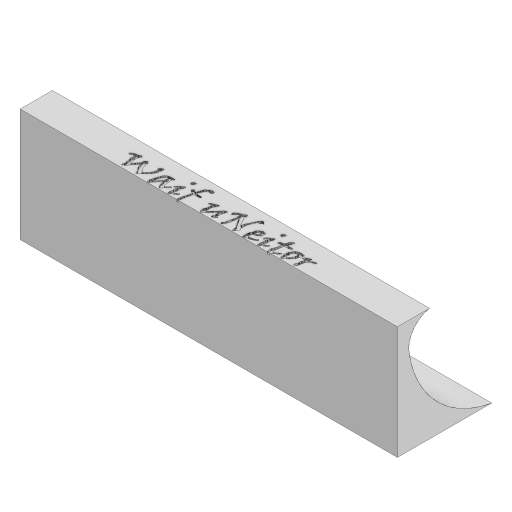
# Autodesk Inventor part: aaaaaa
Saved by Autodesk Inventor 2024.3 (Build 283343000, 343)
## iProperties
Created: 2025-09-24
Part Number: aaaaaa
Material: Generic
Document SubType Name: Modeling
Designer: danie
Density: 1 g/cm^3
Appearance: Default
Author: danie
Autodesk Inventor part; units mm, degrees
(part 1 of 3)
ref_plane "YZ Plane" through (0, 0, 0) normal (1, 0, 0) x (0, 1, 0)
ref_plane "XZ Plane" through (0, 0, 0) normal (0, 1, 0) x (-1, 0, 0)
ref_plane "XY Plane" through (0, 0, 0) normal (0, 0, 1) x (1, 0, 0)
sketch "Sketch1" plane through (0, 0, 0) normal (0, 1, 0) x (-1, 0, 0)
  line L0 (0, 0) -> (200, 0)
  line L1 (200, 0) -> (200, -50)
  line L2 (200, -50) -> (0, -50)
  line L3 (0, -50) -> (0, 0)
  dimension "d0" = 200
  dimension "d1" = 50
  constraints: 8 end point, 2 parallel, 1 horizontal, 1 perpendicular
  measures "d0" distance of L1.end L2.end
  measures "d1" distance of L0.end L1.end
extrude "Extrusion1" add sketch "Sketch1" along normal blind 60
sketch "Sketch2" plane through (0, 0, 0) normal (1, 0, 0) x (0, 0, -1)
  line L0 (0, 0) -> (10, 0)
  line L1 (50, 0) -> (0, 0) projected
  line L2 (10, 0) -> (10, 42.4907)
  line L3 (50, 60) -> (0, 60) projected
  line L4 (0, 60) -> (10, 60)
  line L5 (0, 60) -> (0, 0)
  line L6 (50, 0) -> (50, 60) projected
  line L7 (50, 0) -> (10, 0)
  line L8 (10, 36.0626) -> (10, 0)
  line L9 (50, 0) -> (10, 0)
  line L10 (10, 0) -> (10, 60)
  line L11 (50, 0) -> (5.9553, 46.7873)
  line L12 (5.9553, 46.7873) -> (5.9553, 0)
  line L13 (5.9553, 0) -> (5.9553, 60)
  arc A0 (5.9553, 46.7873) -> (50, 0) centre (58.9478, 52.5484) ccw
  arc A1 (21.7431, 60) -> (5.9553, 46.7873) centre (19.3779, 46.7873) ccw
  line L14 (10, 60) -> (50, 60)
  line L15 (50, 60) -> (50, 0)
  point P0 (17.0127, 60)
  dimension "d4" = 10
  constraints: 26 end point, 7 collinear, 7 point on line, 4 point on circle, 3 perpendicular, 2 centre point, 1 tangent
  measures "d4" distance of L0.start L0.end
extrude "Extrusion2" cut sketch "Sketch2" against normal blind 205.75 contours A1 L10 L11 | L11 L2 A0 | L11 L10 A1 L3 L6 | A0 L2 L11
sketch "Sketch3" plane through (0, 60, 0) normal (0, 1, 0) x (1, 0, 0)
  line L0 (-151.1336, 0) -> (-72.8185, 0)
  line L1 (-200, 0) -> (0, 0) projected
  line L2 (-151.1336, 0) -> (-151.1336, 4.8193)
  line L3 (-151.1336, 1.3121) -> (-68.8391, 1.3121)
  spline S0 degree 2 poles (-146.2846, 10.7529) (-145.9785, 10.6182) (-145.8927, 10.508) knots 0 0 0 1 1 1
  line L4 (-145.8927, 10.508) -> (-145.8683, 10.2753)
  line L5 (-145.8683, 10.2753) -> (-145.5376, 10.2019)
  spline S1 degree 2 poles (-145.5376, 10.2019) (-145.5989, 10.1284) (-146.0029, 9.81) knots 0 0 0 1 1 1
  line L6 (-146.0029, 9.81) -> (-146.1499, 9.4549)
  line L7 (-146.1499, 9.4549) -> (-146.1499, 9.259)
  line L8 (-146.1499, 9.259) -> (-146.1009, 9.1121)
  line L9 (-146.1009, 9.1121) -> (-146.3458, 8.6468)
  line L10 (-146.3458, 8.6468) -> (-146.3213, 8.1447)
  line L11 (-146.3213, 8.1447) -> (-146.4193, 7.8998)
  line L12 (-146.4193, 7.8998) -> (-146.5295, 7.2019)
  line L13 (-146.5295, 7.2019) -> (-146.4193, 6.9815)
  line L14 (-146.4193, 6.9815) -> (-146.456, 6.7121)
  line L15 (-146.456, 6.7121) -> (-146.4193, 6.6386)
  line L16 (-146.4193, 6.6386) -> (-146.5295, 6.5651)
  line L17 (-146.5295, 6.5651) -> (-146.1744, 5.2549)
  line L18 (-146.1744, 5.2549) -> (-146.2601, 5.1937)
  line L19 (-146.2601, 5.1937) -> (-145.758, 4.3121)
  line L20 (-145.758, 4.3121) -> (-145.5376, 4.4223)
  line L21 (-145.5376, 4.4223) -> (-145.5131, 4.557)
  spline S2 degree 2 poles (-145.5131, 4.557) (-145.5131, 4.6182) (-145.3662, 4.8141) (-145.1213, 5.01) knots 0 0 0 1 2 2 2
  spline S3 degree 2 poles (-145.1213, 5.01) (-145.1213, 5.0835) (-144.9009, 5.4019) knots 0 0 0 1 1 1
  line L22 (-144.9009, 5.4019) -> (-144.8764, 5.3774)
  line L23 (-144.8764, 5.3774) -> (-144.7662, 5.4753)
  line L24 (-144.7662, 5.4753) -> (-144.7295, 5.61)
  line L25 (-144.7295, 5.61) -> (-144.5948, 5.7325)
  line L26 (-144.5948, 5.7325) -> (-144.6193, 5.9651)
  spline S4 degree 2 poles (-144.6193, 5.9651) (-144.5091, 5.9896) (-144.2029, 6.1488) knots 0 0 0 1 1 1
  line L27 (-144.2029, 6.1488) -> (-144.1172, 6.308)
  line L28 (-144.1172, 6.308) -> (-144.056, 6.308)
  spline S5 degree 2 poles (-144.056, 6.308) (-143.9336, 6.5406) (-143.7009, 6.7121) knots 0 0 0 1 1 1
  line L29 (-143.7009, 6.7121) -> (-143.6764, 6.8835)
  spline S6 degree 2 poles (-143.6764, 6.8835) (-143.6029, 6.9447) (-143.3213, 7.3121) knots 0 0 0 1 1 1
  line L30 (-143.3213, 7.3121) -> (-143.3458, 7.3488)
  line L31 (-143.3458, 7.3488) -> (-143.2601, 7.4223)
  line L32 (-143.2601, 7.4223) -> (-143.2601, 7.7039)
  line L33 (-143.2601, 7.7039) -> (-143.1499, 8.059)
  line L34 (-143.1499, 8.059) -> (-143.2846, 8.3406)
  line L35 (-143.2846, 8.3406) -> (-143.2601, 8.6223)
  line L36 (-143.2601, 8.6223) -> (-143.3458, 8.7815)
  spline S7 degree 2 poles (-143.3458, 8.7815) (-143.3336, 8.8427) (-143.1744, 9.0019) knots 0 0 0 1 1 1
  line L37 (-143.1744, 9.0019) -> (-143.0642, 9.0019)
  line L38 (-143.0642, 9.0019) -> (-142.8683, 9.1121)
  line L39 (-142.8683, 9.1121) -> (-142.8683, 9.3202)
  line L40 (-142.8683, 9.3202) -> (-142.6846, 9.4182)
  line L41 (-142.6846, 9.4182) -> (-142.5376, 9.357)
  spline S8 degree 2 poles (-142.5376, 9.357) (-142.4274, 9.5406) (-142.3417, 9.6386) knots 0 0 0 1 1 1
  line L42 (-142.3417, 9.6386) -> (-141.9866, 9.7488)
  line L43 (-141.9866, 9.7488) -> (-141.705, 9.6019)
  line L44 (-141.705, 9.6019) -> (-141.5091, 9.0019)
  line L45 (-141.5091, 9.0019) -> (-141.1295, 8.757)
  line L46 (-141.1295, 8.757) -> (-141.0683, 7.9488)
  line L47 (-141.0683, 7.9488) -> (-141.0315, 7.8019)
  line L48 (-141.0315, 7.8019) -> (-141.0683, 7.6182)
  line L49 (-141.0683, 7.6182) -> (-140.958, 7.5202)
  line L50 (-140.958, 7.5202) -> (-140.8846, 7.0672)
  line L51 (-140.8846, 7.0672) -> (-140.7131, 6.5039)
  line L52 (-140.7131, 6.5039) -> (-140.6764, 6.308)
  line L53 (-140.6764, 6.308) -> (-140.0152, 4.9733)
  line L54 (-140.0152, 4.9733) -> (-139.5866, 4.2386)
  line L55 (-139.5866, 4.2386) -> (-139.2927, 4.1406)
  line L56 (-139.2927, 4.1406) -> (-139.256, 3.7611)
  line L57 (-139.256, 3.7611) -> (-139.0968, 3.6753)
  line L58 (-139.0968, 3.6753) -> (-139.0111, 3.6753)
  line L59 (-139.0111, 3.6753) -> (-138.8397, 3.5039)
  spline S9 degree 2 poles (-138.8397, 3.5039) (-138.7662, 3.4304) (-138.5948, 3.1121) knots 0 0 0 1 1 1
  line L60 (-138.5948, 3.1121) -> (-138.3744, 3.1488)
  line L61 (-138.3744, 3.1488) -> (-138.2764, 3.357)
  line L62 (-138.2764, 3.357) -> (-138.1295, 3.4549)
  line L63 (-138.1295, 3.4549) -> (-138.0315, 3.6019)
  spline S10 degree 2 poles (-138.0315, 3.6019) (-137.9825, 3.6753) (-137.7376, 3.8957) knots 0 0 0 1 1 1
  line L64 (-137.7376, 3.8957) -> (-137.6764, 3.9202)
  line L65 (-137.6764, 3.9202) -> (-137.5172, 4.1284)
  spline S11 degree 2 poles (-137.5172, 4.1284) (-137.4315, 4.2386) (-137.2601, 4.3366) knots 0 0 0 1 1 1
  line L66 (-137.2601, 4.3366) -> (-137.2111, 4.4835)
  line L67 (-137.2111, 4.4835) -> (-137.0029, 4.6672)
  spline S12 degree 2 poles (-137.0029, 4.6672) (-136.8805, 4.9488) (-136.7213, 5.0835) (-136.5376, 5.157) knots 0 0 0 1 2 2 2
  line L68 (-136.5376, 5.157) -> (-136.4764, 5.3284)
  line L69 (-136.4764, 5.3284) -> (-136.4397, 5.3039)
  line L70 (-136.4397, 5.3039) -> (-136.354, 5.6223)
  spline S13 degree 2 poles (-136.354, 5.6223) (-136.3417, 5.6713) (-136.207, 5.8672) knots 0 0 0 1 1 1
  line L71 (-136.207, 5.8672) -> (-136.1213, 5.8672)
  line L72 (-136.1213, 5.8672) -> (-136.0111, 5.9651)
  line L73 (-136.0111, 5.9651) -> (-135.9499, 6.2835)
  line L74 (-135.9499, 6.2835) -> (-135.705, 6.7488)
  line L75 (-135.705, 6.7488) -> (-135.5948, 6.8468)
  line L76 (-135.5948, 6.8468) -> (-135.6683, 6.9447)
  line L77 (-135.6683, 6.9447) -> (-135.5213, 7.2264)
  line L78 (-135.5213, 7.2264) -> (-135.5213, 7.7039)
  line L79 (-135.5213, 7.7039) -> (-135.4601, 7.7039)
  line L80 (-135.4601, 7.7039) -> (-135.3744, 7.8019)
  line L81 (-135.3744, 7.8019) -> (-135.3131, 7.8019)
  line L82 (-135.3131, 7.8019) -> (-135.3744, 8.3406)
  line L83 (-135.3744, 8.3406) -> (-135.4601, 8.757)
  line L84 (-135.4601, 8.757) -> (-135.9866, 8.757)
  line L85 (-135.9866, 8.757) -> (-136.1213, 9.0386)
  line L86 (-136.1213, 9.0386) -> (-136.0111, 9.1733)
  line L87 (-136.0111, 9.1733) -> (-135.9499, 9.3202)
  line L88 (-135.9499, 9.3202) -> (-135.8274, 9.4549)
  spline S14 degree 2 poles (-135.8274, 9.4549) (-135.7662, 9.5284) (-135.705, 9.6998) knots 0 0 0 1 1 1
  line L89 (-135.705, 9.6998) -> (-135.5703, 9.7855)
  line L90 (-135.5703, 9.7855) -> (-135.5703, 9.9202)
  line L91 (-135.5703, 9.9202) -> (-135.3744, 10.0304)
  line L92 (-135.3744, 10.0304) -> (-135.2887, 9.957)
  line L93 (-135.2887, 9.957) -> (-135.2397, 10.2019)
  spline S15 degree 2 poles (-135.2397, 10.2019) (-134.8601, 10.3855) (-134.7499, 10.4835) knots 0 0 0 1 1 1
  line L94 (-134.7499, 10.4835) -> (-134.505, 10.3733)
  line L95 (-134.505, 10.3733) -> (-134.3213, 10.508)
  line L96 (-134.3213, 10.508) -> (-134.2111, 10.508)
  line L97 (-134.2111, 10.508) -> (-134.0642, 10.2386)
  line L98 (-134.0642, 10.2386) -> (-134.1866, 10.0549)
  line L99 (-134.1866, 10.0549) -> (-134.0642, 9.7488)
  line L100 (-134.0642, 9.7488) -> (-134.0642, 8.6468)
  line L101 (-134.0642, 8.6468) -> (-134.1866, 8.5366)
  line L102 (-134.1866, 8.5366) -> (-134.1499, 8.3651)
  line L103 (-134.1499, 8.3651) -> (-134.1866, 8.0835)
  line L104 (-134.1866, 8.0835) -> (-134.2601, 8.059)
  line L105 (-134.2601, 8.059) -> (-134.3948, 7.4468)
  line L106 (-134.3948, 7.4468) -> (-134.5295, 7.2508)
  spline S16 degree 2 poles (-134.5295, 7.2508) (-134.6029, 7.1406) (-134.6274, 7.0549) knots 0 0 0 1 1 1
  line L107 (-134.6274, 7.0549) -> (-134.6764, 6.81)
  line L108 (-134.6764, 6.81) -> (-134.6764, 6.6753)
  line L109 (-134.6764, 6.6753) -> (-134.958, 6.1488)
  line L110 (-134.958, 6.1488) -> (-135.5213, 5.4753)
  line L111 (-135.5213, 5.4753) -> (-135.4846, 5.3774)
  line L112 (-135.4846, 5.3774) -> (-135.7295, 4.9488)
  line L113 (-135.7295, 4.9488) -> (-136.7948, 3.7855)
  line L114 (-136.7948, 3.7855) -> (-136.9295, 3.6998)
  line L115 (-136.9295, 3.6998) -> (-137.1499, 3.4304)
  line L116 (-137.1499, 3.4304) -> (-138.7662, 1.6182)
  line L117 (-138.7662, 1.6182) -> (-139.1948, 1.4468)
  line L118 (-139.1948, 1.4468) -> (-139.3785, 1.3121)
  line L119 (-139.3785, 1.3121) -> (-139.5376, 1.3611)
  line L120 (-139.5376, 1.3611) -> (-139.8193, 1.0304)
  line L121 (-139.8193, 1.0304) -> (-139.954, 1.0917)
  line L122 (-139.954, 1.0917) -> (-140.3213, 2.157)
  line L123 (-140.3213, 2.157) -> (-140.3213, 2.3406)
  line L124 (-140.3213, 2.3406) -> (-140.407, 2.4141)
  spline S17 degree 2 poles (-140.407, 2.4141) (-140.456, 2.4508) (-140.5662, 2.6957) knots 0 0 0 1 1 1
  line L125 (-140.5662, 2.6957) -> (-140.5907, 2.6957)
  line L126 (-140.5907, 2.6957) -> (-141.0927, 3.3202)
  line L127 (-141.0927, 3.3202) -> (-141.0927, 3.5406)
  line L128 (-141.0927, 3.5406) -> (-141.4234, 3.7855)
  spline S18 degree 2 poles (-141.4234, 3.7855) (-141.5825, 3.9447) (-141.7662, 4.0917) knots 0 0 0 1 1 1
  line L129 (-141.7662, 4.0917) -> (-141.8397, 4.459)
  line L130 (-141.8397, 4.459) -> (-142.0111, 4.5937)
  line L131 (-142.0111, 4.5937) -> (-141.9009, 4.7651)
  line L132 (-141.9009, 4.7651) -> (-142.1458, 5.059)
  line L133 (-142.1458, 5.059) -> (-142.6478, 6.3937)
  line L134 (-142.6478, 6.3937) -> (-142.6234, 6.4549)
  line L135 (-142.6234, 6.4549) -> (-142.6478, 6.6753)
  line L136 (-142.6478, 6.6753) -> (-142.9662, 6.6386)
  line L137 (-142.9662, 6.6386) -> (-143.1131, 6.1733)
  line L138 (-143.1131, 6.1733) -> (-143.4193, 5.8917)
  line L139 (-143.4193, 5.8917) -> (-143.3948, 5.8304)
  line L140 (-143.3948, 5.8304) -> (-144.3744, 4.6917)
  line L141 (-144.3744, 4.6917) -> (-145.1825, 3.5039)
  line L142 (-145.1825, 3.5039) -> (-145.256, 3.3325)
  spline S19 degree 2 poles (-145.256, 3.3325) (-145.2927, 3.259) (-145.5131, 3.0386) (-145.6723, 2.9284) knots 0 0 0 1 2 2 2
  line L143 (-145.6723, 2.9284) -> (-145.7213, 2.6957)
  line L144 (-145.7213, 2.6957) -> (-145.9295, 2.5121)
  line L145 (-145.9295, 2.5121) -> (-145.954, 2.3651)
  line L146 (-145.954, 2.3651) -> (-146.1009, 2.3039)
  line L147 (-146.1009, 2.3039) -> (-146.1009, 2.1202)
  line L148 (-146.1009, 2.1202) -> (-146.3948, 1.8386)
  line L149 (-146.3948, 1.8386) -> (-146.8111, 1.8386)
  line L150 (-146.8111, 1.8386) -> (-146.8723, 1.6182)
  line L151 (-146.8723, 1.6182) -> (-147.0927, 1.4835)
  spline S20 degree 2 poles (-147.0927, 1.4835) (-147.2519, 1.2876) (-147.3989, 1.1774) knots 0 0 0 1 1 1
  line L152 (-147.3989, 1.1774) -> (-147.656, 1.3978)
  spline S21 degree 2 poles (-147.656, 1.3978) (-147.6927, 1.4468) (-147.7662, 1.6182) knots 0 0 0 1 1 1
  line L153 (-147.7662, 1.6182) -> (-147.5948, 1.9855)
  spline S22 degree 2 poles (-147.5948, 1.9855) (-147.558, 2.1202) (-147.3989, 2.5121) knots 0 0 0 1 1 1
  line L154 (-147.3989, 2.5121) -> (-147.4846, 2.6957)
  line L155 (-147.4846, 2.6957) -> (-147.4478, 2.7202)
  line L156 (-147.4478, 2.7202) -> (-147.4478, 2.9284)
  line L157 (-147.4478, 2.9284) -> (-147.3744, 3.0019)
  line L158 (-147.3744, 3.0019) -> (-147.4846, 3.3937)
  line L159 (-147.4846, 3.3937) -> (-147.3989, 3.6141)
  line L160 (-147.3989, 3.6141) -> (-147.558, 3.9202)
  line L161 (-147.558, 3.9202) -> (-147.5091, 4.0304)
  line L162 (-147.5091, 4.0304) -> (-147.6193, 4.0917)
  line L163 (-147.6193, 4.0917) -> (-147.6193, 4.3121)
  line L164 (-147.6193, 4.3121) -> (-147.9009, 5.8304)
  line L165 (-147.9009, 5.8304) -> (-147.9009, 6.0753)
  line L166 (-147.9009, 6.0753) -> (-148.2315, 6.5651)
  line L167 (-148.2315, 6.5651) -> (-148.2315, 6.81)
  line L168 (-148.2315, 6.81) -> (-148.0111, 7.2753)
  line L169 (-148.0111, 7.2753) -> (-148.0111, 7.3121)
  line L170 (-148.0111, 7.3121) -> (-148.1213, 7.4223)
  line L171 (-148.1213, 7.4223) -> (-147.9744, 8.1447)
  spline S23 degree 2 poles (-147.9744, 8.1447) (-147.8887, 8.4998) (-147.8397, 8.5855) knots 0 0 0 1 1 1
  line L172 (-147.8397, 8.5855) -> (-148.0356, 9.0386)
  line L173 (-148.0356, 9.0386) -> (-149.0642, 8.8304)
  line L174 (-149.0642, 8.8304) -> (-149.4315, 8.6835)
  line L175 (-149.4315, 8.6835) -> (-149.6274, 8.6835)
  line L176 (-149.6274, 8.6835) -> (-149.8723, 8.5366)
  line L177 (-149.8723, 8.5366) -> (-150.2274, 8.2182)
  line L178 (-150.2274, 8.2182) -> (-150.705, 8.2549)
  line L179 (-150.705, 8.2549) -> (-150.9009, 8.757)
  line L180 (-150.9009, 8.757) -> (-150.7662, 8.7815)
  line L181 (-150.7662, 8.7815) -> (-150.5825, 9.0141)
  spline S24 degree 2 poles (-150.5825, 9.0141) (-150.4846, 9.1366) (-150.3744, 9.1978) (-150.2029, 9.3202) knots 0 0 0 1 2 2 2
  line L182 (-150.2029, 9.3202) -> (-150.0683, 9.3202)
  spline S25 degree 2 poles (-150.0683, 9.3202) (-149.9703, 9.4427) (-149.5662, 9.6386) knots 0 0 0 1 1 1
  line L183 (-149.5662, 9.6386) -> (-149.5295, 9.7488)
  line L184 (-149.5295, 9.7488) -> (-149.1499, 9.7855)
  line L185 (-149.1499, 9.7855) -> (-148.8805, 9.9202)
  line L186 (-148.8805, 9.9202) -> (-148.7091, 9.9202)
  line L187 (-148.7091, 9.9202) -> (-148.6478, 9.8835)
  spline S26 degree 2 poles (-148.6478, 9.8835) (-148.6356, 9.9447) (-148.5131, 10.0304) knots 0 0 0 1 1 1
  line L188 (-148.5131, 10.0304) -> (-148.4274, 9.8345)
  line L189 (-148.4274, 9.8345) -> (-147.8397, 10.0549)
  line L190 (-147.8397, 10.0549) -> (-147.8397, 10.0917)
  line L191 (-147.8397, 10.0917) -> (-147.5948, 10.0549)
  line L192 (-147.5948, 10.0549) -> (-147.4478, 10.0917)
  spline S27 degree 2 poles (-147.4478, 10.0917) (-147.3989, 10.1406) (-147.0927, 10.3733) knots 0 0 0 1 1 1
  line L193 (-147.0927, 10.3733) -> (-146.7866, 10.3366)
  spline S28 degree 2 poles (-146.7866, 10.3366) (-146.7499, 10.4468) (-146.5662, 10.6672) knots 0 0 0 1 1 1
  line L194 (-146.5662, 10.6672) -> (-146.2846, 10.7529)
  spline S29 degree 2 poles (-127.5621, 8.757) (-127.5131, 8.7692) (-127.0234, 8.708) (-126.9621, 8.6345) knots 0 0 0 1 2 2 2
  line L195 (-126.9621, 8.6345) -> (-126.705, 8.6957)
  line L196 (-126.705, 8.6957) -> (-126.558, 8.6835)
  line L197 (-126.558, 8.6835) -> (-126.4478, 8.4753)
  line L198 (-126.4478, 8.4753) -> (-126.4601, 8.3284)
  spline S30 degree 2 poles (-126.4601, 8.3284) (-126.6193, 8.2059) (-126.6682, 8.059) knots 0 0 0 1 1 1
  line L199 (-126.6682, 8.059) -> (-126.7417, 8.059)
  line L200 (-126.7417, 8.059) -> (-126.8274, 7.9611)
  spline S31 degree 2 poles (-126.8274, 7.9611) (-126.8642, 7.9243) (-127.1458, 7.8386) knots 0 0 0 1 1 1
  line L201 (-127.1458, 7.8386) -> (-127.158, 6.4304)
  line L202 (-127.158, 6.4304) -> (-127.0356, 5.6957)
  line L203 (-127.0356, 5.6957) -> (-127.0234, 4.9488)
  line L204 (-127.0234, 4.9488) -> (-126.9131, 4.0304)
  line L205 (-126.9131, 4.0304) -> (-126.4356, 2.7202)
  spline S32 degree 2 poles (-126.4356, 2.7202) (-126.3009, 2.5733) (-126.2642, 2.4998) knots 0 0 0 1 1 1
  spline S33 degree 2 poles (-126.2642, 2.4998) (-125.8846, 2.708) (-125.7866, 2.708) knots 0 0 0 1 1 1
  spline S34 degree 2 poles (-125.7866, 2.708) (-125.4682, 3.0631) (-125.3825, 3.0753) knots 0 0 0 1 1 1
  line L206 (-125.3825, 3.0753) -> (-125.3825, 3.1611)
  line L207 (-125.3825, 3.1611) -> (-124.5254, 3.8957)
  line L208 (-124.5254, 3.8957) -> (-124.5009, 4.0304)
  spline S35 degree 2 poles (-124.5009, 4.0304) (-124.4274, 4.0427) (-124.1825, 4.3243) knots 0 0 0 1 1 1
  line L209 (-124.1825, 4.3243) -> (-123.9009, 4.2631)
  line L210 (-123.9009, 4.2631) -> (-123.7417, 3.9202)
  line L211 (-123.7417, 3.9202) -> (-123.8029, 3.6264)
  line L212 (-123.8029, 3.6264) -> (-123.9621, 3.6876)
  line L213 (-123.9621, 3.6876) -> (-124.0356, 3.5162)
  line L214 (-124.0356, 3.5162) -> (-124.1825, 3.5162)
  spline S36 degree 2 poles (-124.1825, 3.5162) (-124.2682, 3.2957) (-124.4274, 3.1488) knots 0 0 0 1 1 1
  line L215 (-124.4274, 3.1488) -> (-124.4274, 3.0631)
  line L216 (-124.4274, 3.0631) -> (-124.8438, 2.6835)
  line L217 (-124.8438, 2.6835) -> (-124.9295, 2.4753)
  spline S37 degree 2 poles (-124.9295, 2.4753) (-125.0642, 2.3774) (-125.407, 2.2182) knots 0 0 0 1 1 1
  line L218 (-125.407, 2.2182) -> (-125.4682, 2.0957)
  line L219 (-125.4682, 2.0957) -> (-125.4805, 2.1447)
  line L220 (-125.4805, 2.1447) -> (-125.5785, 1.9855)
  line L221 (-125.5785, 1.9855) -> (-125.7866, 1.9243)
  line L222 (-125.7866, 1.9243) -> (-125.8111, 1.8141)
  line L223 (-125.8111, 1.8141) -> (-125.9213, 1.8141)
  line L224 (-125.9213, 1.8141) -> (-125.8723, 1.7039)
  line L225 (-125.8723, 1.7039) -> (-125.9948, 1.459)
  line L226 (-125.9948, 1.459) -> (-126.105, 1.4345)
  spline S38 degree 2 poles (-126.105, 1.4345) (-126.0927, 1.3121) (-126.3621, 0.9815) knots 0 0 0 1 1 1
  line L227 (-126.3621, 0.9815) -> (-126.7172, 0.9692)
  line L228 (-126.7172, 0.9692) -> (-126.7907, 0.7488)
  line L229 (-126.7907, 0.7488) -> (-127.0111, 0.6876)
  spline S39 degree 2 poles (-127.0111, 0.6876) (-127.256, 0.7611) (-127.4152, 1.0059) knots 0 0 0 1 1 1
  line L230 (-127.4152, 1.0059) -> (-127.9172, 1.8264)
  line L231 (-127.9172, 1.8264) -> (-128.407, 2.9162)
  line L232 (-128.407, 2.9162) -> (-128.358, 3.3202)
  line L233 (-128.358, 3.3202) -> (-128.4682, 3.6753)
  line L234 (-128.4682, 3.6753) -> (-128.3948, 3.6876)
  spline S40 degree 2 poles (-128.3948, 3.6876) (-128.6152, 4.1284) (-128.6152, 4.3488) knots 0 0 0 1 1 1
  line L235 (-128.6152, 4.3488) -> (-128.5785, 4.6304)
  line L236 (-128.5785, 4.6304) -> (-128.8111, 4.7774)
  line L237 (-128.8111, 4.7774) -> (-128.9703, 4.6794)
  line L238 (-128.9703, 4.6794) -> (-128.9703, 4.7162)
  line L239 (-128.9703, 4.7162) -> (-129.0438, 4.6794)
  line L240 (-129.0438, 4.6794) -> (-129.2519, 4.1529)
  line L241 (-129.2519, 4.1529) -> (-129.3499, 4.2019)
  line L242 (-129.3499, 4.2019) -> (-129.3866, 4.0917)
  line L243 (-129.3866, 4.0917) -> (-129.4601, 4.1284)
  line L244 (-129.4601, 4.1284) -> (-129.4601, 4.0549)
  line L245 (-129.4601, 4.0549) -> (-129.4968, 4.0549)
  spline S41 degree 2 poles (-129.4968, 4.0549) (-129.4968, 4.0182) (-129.7172, 3.6753) knots 0 0 0 1 1 1
  line L246 (-129.7172, 3.6753) -> (-129.7662, 3.6998)
  line L247 (-129.7662, 3.6998) -> (-129.8152, 3.3815)
  line L248 (-129.8152, 3.3815) -> (-129.9744, 3.2957)
  spline S42 degree 2 poles (-129.9744, 3.2957) (-130.1336, 3.21) (-130.1825, 3.0998) knots 0 0 0 1 1 1
  line L249 (-130.1825, 3.0998) -> (-130.2438, 2.9406)
  line L250 (-130.2438, 2.9406) -> (-130.1703, 2.8549)
  line L251 (-130.1703, 2.8549) -> (-130.354, 2.7937)
  line L252 (-130.354, 2.7937) -> (-130.4274, 2.4753)
  line L253 (-130.4274, 2.4753) -> (-130.5499, 2.4141)
  line L254 (-130.5499, 2.4141) -> (-130.5131, 2.3529)
  spline S43 degree 2 poles (-130.5131, 2.3529) (-130.6968, 2.2182) (-130.807, 2.1692) knots 0 0 0 1 1 1
  line L255 (-130.807, 2.1692) -> (-130.8805, 2.059)
  line L256 (-130.8805, 2.059) -> (-130.9417, 2.1447)
  line L257 (-130.9417, 2.1447) -> (-131.0519, 1.8753)
  line L258 (-131.0519, 1.8753) -> (-131.1376, 1.8753)
  line L259 (-131.1376, 1.8753) -> (-131.2723, 1.4345)
  line L260 (-131.2723, 1.4345) -> (-131.407, 1.3855)
  line L261 (-131.407, 1.3855) -> (-131.4193, 1.1651)
  line L262 (-131.4193, 1.1651) -> (-131.6397, 1.1651)
  line L263 (-131.6397, 1.1651) -> (-131.8601, 0.6631)
  line L264 (-131.8601, 0.6631) -> (-131.9703, 0.5896)
  line L265 (-131.9703, 0.5896) -> (-132.056, 0.5896)
  line L266 (-132.056, 0.5896) -> (-132.0805, 0.4427)
  line L267 (-132.0805, 0.4427) -> (-132.5703, 0.259)
  line L268 (-132.5703, 0.259) -> (-133.0846, 0.2468)
  line L269 (-133.0846, 0.2468) -> (-133.305, 1.6794)
  line L270 (-133.305, 1.6794) -> (-133.207, 1.8753)
  line L271 (-133.207, 1.8753) -> (-133.1825, 2.0223)
  spline S44 degree 2 poles (-133.1825, 2.0223) (-133.1825, 2.0835) (-132.9989, 2.4753) knots 0 0 0 1 1 1
  line L272 (-132.9989, 2.4753) -> (-133.0356, 2.5855)
  spline S45 degree 2 poles (-133.0356, 2.5855) (-132.9009, 2.9039) (-132.8519, 2.9529) knots 0 0 0 1 1 1
  line L273 (-132.8519, 2.9529) -> (-132.9131, 2.9896)
  line L274 (-132.9131, 2.9896) -> (-132.7662, 3.357)
  line L275 (-132.7662, 3.357) -> (-132.7662, 3.5039)
  spline S46 degree 2 poles (-132.7662, 3.5039) (-132.754, 3.5651) (-132.6438, 3.7855) knots 0 0 0 1 1 1
  spline S47 degree 2 poles (-132.6438, 3.7855) (-132.705, 4.1529) (-132.7662, 4.2019) knots 0 0 0 1 1 1
  line L276 (-132.7662, 4.2019) -> (-132.705, 4.3121)
  line L277 (-132.705, 4.3121) -> (-132.5091, 4.2753)
  spline S48 degree 2 poles (-132.5091, 4.2753) (-132.3376, 4.508) (-132.2887, 4.5325) knots 0 0 0 1 1 1
  line L278 (-132.2887, 4.5325) -> (-132.2397, 4.6672)
  line L279 (-132.2397, 4.6672) -> (-132.2152, 4.6672)
  line L280 (-132.2152, 4.6672) -> (-132.3254, 4.8264)
  line L281 (-132.3254, 4.8264) -> (-132.2274, 5.2304)
  line L282 (-132.2274, 5.2304) -> (-132.1662, 5.1937)
  spline S49 degree 2 poles (-132.1662, 5.1937) (-132.0805, 5.4264) (-132.056, 5.4264) knots 0 0 0 1 1 1
  line L283 (-132.056, 5.4264) -> (-132.0805, 5.6345)
  line L284 (-132.0805, 5.6345) -> (-131.8723, 6.0264)
  line L285 (-131.8723, 6.0264) -> (-131.8723, 6.1243)
  line L286 (-131.8723, 6.1243) -> (-131.9213, 6.2223)
  line L287 (-131.9213, 6.2223) -> (-131.6029, 6.8835)
  line L288 (-131.6029, 6.8835) -> (-131.2478, 7.3733)
  spline S50 degree 2 poles (-131.2478, 7.3733) (-131.0642, 7.5325) (-130.9417, 7.7284) knots 0 0 0 1 1 1
  line L289 (-130.9417, 7.7284) -> (-130.6723, 7.8386)
  line L290 (-130.6723, 7.8386) -> (-130.3172, 8.2059)
  line L291 (-130.3172, 8.2059) -> (-129.9744, 8.4141)
  line L292 (-129.9744, 8.4141) -> (-129.7662, 8.4141)
  line L293 (-129.7662, 8.4141) -> (-129.607, 8.4631)
  line L294 (-129.607, 8.4631) -> (-129.3744, 8.4631)
  line L295 (-129.3744, 8.4631) -> (-129.2642, 8.6345)
  line L296 (-129.2642, 8.6345) -> (-129.0438, 8.6223)
  line L297 (-129.0438, 8.6223) -> (-128.8234, 8.6223)
  line L298 (-128.8234, 8.6223) -> (-128.8234, 8.6835)
  spline S51 degree 2 poles (-128.8234, 8.6835) (-128.7376, 8.6713) (-128.6274, 8.5978) knots 0 0 0 1 1 1
  line L299 (-128.6274, 8.5978) -> (-128.3948, 8.6957)
  line L300 (-128.3948, 8.6957) -> (-128.2111, 8.6468)
  line L301 (-128.2111, 8.6468) -> (-128.1744, 8.708)
  line L302 (-128.1744, 8.708) -> (-127.9907, 8.6468)
  line L303 (-127.9907, 8.6468) -> (-127.5621, 8.757)
  line L304 (-129.5213, 7.557) -> (-129.7172, 7.5202)
  line L305 (-129.7172, 7.5202) -> (-129.9499, 7.5447)
  line L306 (-129.9499, 7.5447) -> (-130.0234, 7.41)
  line L307 (-130.0234, 7.41) -> (-130.0234, 7.2876)
  spline S52 degree 2 poles (-130.0234, 7.2876) (-130.1458, 7.2264) (-130.2927, 7.1896) knots 0 0 0 1 1 1
  line L308 (-130.2927, 7.1896) -> (-130.4274, 6.8468)
  spline S53 degree 2 poles (-130.4274, 6.8468) (-130.5254, 6.3937) (-130.5499, 6.3815) knots 0 0 0 1 1 1
  line L309 (-130.5499, 6.3815) -> (-130.6234, 6.3815)
  line L310 (-130.6234, 6.3815) -> (-130.7336, 6.1243)
  line L311 (-130.7336, 6.1243) -> (-130.7825, 5.9162)
  spline S54 degree 2 poles (-130.7825, 5.9162) (-130.807, 5.8182) (-130.9417, 5.757) knots 0 0 0 1 1 1
  line L312 (-130.9417, 5.757) -> (-131.0152, 5.4876)
  line L313 (-131.0152, 5.4876) -> (-131.1376, 5.2672)
  spline S55 degree 2 poles (-131.1376, 5.2672) (-131.2111, 5.1325) (-131.2111, 4.9978) knots 0 0 0 1 1 1
  line L314 (-131.2111, 4.9978) -> (-131.2111, 4.9366)
  line L315 (-131.2111, 4.9366) -> (-131.2846, 4.9978)
  line L316 (-131.2846, 4.9978) -> (-131.2846, 4.8753)
  line L317 (-131.2846, 4.8753) -> (-131.3213, 4.8753)
  line L318 (-131.3213, 4.8753) -> (-131.3091, 4.7896)
  line L319 (-131.3091, 4.7896) -> (-131.3703, 4.6672)
  line L320 (-131.3703, 4.6672) -> (-131.4683, 4.2631)
  line L321 (-131.4683, 4.2631) -> (-131.6274, 3.9325)
  line L322 (-131.6274, 3.9325) -> (-131.6519, 3.4794)
  line L323 (-131.6519, 3.4794) -> (-131.7009, 3.4059)
  line L324 (-131.7009, 3.4059) -> (-131.7254, 3.4059)
  line L325 (-131.7254, 3.4059) -> (-131.7621, 3.2713)
  line L326 (-131.7621, 3.2713) -> (-131.7009, 3.21)
  line L327 (-131.7009, 3.21) -> (-131.7744, 2.9284)
  line L328 (-131.7744, 2.9284) -> (-131.8111, 2.9284)
  line L329 (-131.8111, 2.9284) -> (-131.7744, 2.8427)
  line L330 (-131.7744, 2.8427) -> (-131.8846, 2.8427)
  line L331 (-131.8846, 2.8427) -> (-131.8723, 2.2794)
  line L332 (-131.8723, 2.2794) -> (-131.8111, 2.01)
  line L333 (-131.8111, 2.01) -> (-131.7744, 2.01)
  line L334 (-131.7744, 2.01) -> (-131.6029, 2.1692)
  line L335 (-131.6029, 2.1692) -> (-131.1621, 2.7937)
  line L336 (-131.1621, 2.7937) -> (-130.3785, 3.8345)
  line L337 (-130.3785, 3.8345) -> (-130.1458, 4.0794)
  line L338 (-130.1458, 4.0794) -> (-129.6193, 4.9366)
  line L339 (-129.6193, 4.9366) -> (-129.0682, 5.659)
  line L340 (-129.0682, 5.659) -> (-129.0315, 5.8182)
  line L341 (-129.0315, 5.8182) -> (-129.1295, 5.9529)
  line L342 (-129.1295, 5.9529) -> (-128.9336, 6.2957)
  line L343 (-128.9336, 6.2957) -> (-128.8968, 6.5529)
  spline S56 degree 2 poles (-128.8968, 6.5529) (-128.8846, 6.5896) (-128.7621, 6.7488) knots 0 0 0 1 1 1
  line L344 (-128.7621, 6.7488) -> (-128.7499, 7.3611)
  line L345 (-128.7499, 7.3611) -> (-128.958, 7.3733)
  line L346 (-128.958, 7.3733) -> (-129.1172, 7.3733)
  line L347 (-129.1172, 7.3733) -> (-129.3376, 7.5202)
  line L348 (-129.3376, 7.5202) -> (-129.3866, 7.4468)
  line L349 (-129.3866, 7.4468) -> (-129.5213, 7.557)
  line L350 (-120.1662, 7.3611) -> (-120.1907, 7.3611)
  line L351 (-120.1907, 7.3611) -> (-120.2519, 6.9692)
  line L352 (-120.2519, 6.9692) -> (-120.1907, 6.9202)
  line L353 (-120.1907, 6.9202) -> (-120.3009, 6.6386)
  line L354 (-120.3009, 6.6386) -> (-120.3376, 6.6876)
  line L355 (-120.3376, 6.6876) -> (-120.3376, 6.5774)
  spline S57 degree 2 poles (-120.3376, 6.5774) (-120.3376, 6.2468) (-120.607, 5.9406) knots 0 0 0 1 1 1
  line L356 (-120.607, 5.9406) -> (-120.558, 5.9406)
  line L357 (-120.558, 5.9406) -> (-120.558, 5.8059)
  line L358 (-120.558, 5.8059) -> (-120.5825, 5.8059)
  line L359 (-120.5825, 5.8059) -> (-120.558, 4.9121)
  line L360 (-120.558, 4.9121) -> (-120.607, 4.8141)
  line L361 (-120.607, 4.8141) -> (-120.5825, 4.6672)
  line L362 (-120.5825, 4.6672) -> (-120.6927, 4.1162)
  line L363 (-120.6927, 4.1162) -> (-120.656, 4.1162)
  spline S58 degree 2 poles (-120.656, 4.1162) (-120.656, 3.957) (-120.7295, 3.6753) knots 0 0 0 1 1 1
  line L364 (-120.7295, 3.6753) -> (-120.8029, 3.4794)
  line L365 (-120.8029, 3.4794) -> (-120.8887, 2.4631)
  spline S59 degree 2 poles (-120.8887, 2.4631) (-120.9254, 2.3162) (-120.9254, 2.2917) knots 0 0 0 1 1 1
  spline S60 degree 2 poles (-120.9254, 2.2917) (-120.9254, 2.157) (-120.8029, 2.157) knots 0 0 0 1 1 1
  spline S61 degree 2 poles (-120.8029, 2.157) (-120.656, 2.157) (-120.4846, 2.2672) knots 0 0 0 1 1 1
  line L366 (-120.4846, 2.2672) -> (-119.9948, 2.5978)
  spline S62 degree 2 poles (-119.9948, 2.5978) (-119.7866, 2.8549) (-119.6887, 2.8549) knots 0 0 0 1 1 1
  line L367 (-119.6887, 2.8549) -> (-119.6519, 2.8549)
  spline S63 degree 2 poles (-119.6519, 2.8549) (-119.5172, 2.9162) (-119.2968, 3.1978) (-119.2356, 3.2223) knots 0 0 0 1 2 2 2
  spline S64 degree 2 poles (-119.2356, 3.2223) (-119.1131, 3.4304) (-119.0274, 3.4304) knots 0 0 0 1 1 1
  spline S65 degree 2 poles (-119.0274, 3.4304) (-119.0152, 3.4304) (-118.9172, 3.3937) (-118.6846, 3.357) knots 0 0 0 1 2 2 2
  line L368 (-118.6846, 3.357) -> (-118.6234, 3.1488)
  spline S66 degree 2 poles (-118.6234, 3.1488) (-118.6234, 2.9774) (-118.8682, 2.5243) (-119.0152, 2.2304) (-119.2601, 2.1447) knots 0 0 0 1 2 3 3 3
  line L369 (-119.2601, 2.1447) -> (-119.2601, 2.0835)
  line L370 (-119.2601, 2.0835) -> (-119.3703, 2.1202)
  line L371 (-119.3703, 2.1202) -> (-119.3703, 2.01)
  line L372 (-119.3703, 2.01) -> (-119.4315, 2.01)
  spline S67 degree 2 poles (-119.4315, 2.01) (-119.456, 1.8019) (-119.6519, 1.7774) knots 0 0 0 1 1 1
  line L373 (-119.6519, 1.7774) -> (-119.6519, 1.7284)
  line L374 (-119.6519, 1.7284) -> (-119.8601, 1.7284)
  line L375 (-119.8601, 1.7284) -> (-119.8601, 1.7039)
  line L376 (-119.8601, 1.7039) -> (-119.9336, 1.7039)
  line L377 (-119.9336, 1.7039) -> (-120.1295, 1.557)
  line L378 (-120.1295, 1.557) -> (-120.1907, 1.557)
  line L379 (-120.1907, 1.557) -> (-120.3009, 1.4223)
  line L380 (-120.3009, 1.4223) -> (-120.607, 1.3733)
  spline S68 degree 2 poles (-120.607, 1.3733) (-120.656, 1.2876) (-120.754, 1.2876) knots 0 0 0 1 1 1
  line L381 (-120.754, 1.2876) -> (-121.1458, 1.0059)
  line L382 (-121.1458, 1.0059) -> (-121.1458, 0.9447)
  line L383 (-121.1458, 0.9447) -> (-121.3295, 0.9692)
  line L384 (-121.3295, 0.9692) -> (-121.2805, 0.8957)
  line L385 (-121.2805, 0.8957) -> (-121.5254, 0.8345)
  line L386 (-121.5254, 0.8345) -> (-121.5254, 0.7978)
  line L387 (-121.5254, 0.7978) -> (-121.6356, 0.7978)
  line L388 (-121.6356, 0.7978) -> (-121.6356, 0.6876)
  line L389 (-121.6356, 0.6876) -> (-121.7458, 0.6141)
  line L390 (-121.7458, 0.6141) -> (-121.7825, 0.6141)
  line L391 (-121.7825, 0.6141) -> (-121.7825, 0.5896)
  spline S69 degree 2 poles (-121.7825, 0.5896) (-121.8805, 0.308) (-122.0642, 0.308) knots 0 0 0 1 1 1
  line L392 (-122.0642, 0.308) -> (-122.1621, 0.3325)
  spline S70 degree 2 poles (-122.1621, 0.3325) (-122.2601, 0.6141) (-122.4805, 0.8957) knots 0 0 0 1 1 1
  spline S71 degree 2 poles (-122.4805, 0.8957) (-122.4193, 1.1406) (-122.4193, 1.2508) knots 0 0 0 1 1 1
  line L393 (-122.4193, 1.2508) -> (-122.4805, 1.557)
  line L394 (-122.4805, 1.557) -> (-122.4805, 1.7284)
  spline S72 degree 2 poles (-122.4805, 1.7284) (-122.4805, 1.9611) (-122.4315, 2.2182) knots 0 0 0 1 1 1
  line L395 (-122.4315, 2.2182) -> (-122.3825, 2.4141)
  line L396 (-122.3825, 2.4141) -> (-122.3825, 2.4508)
  line L397 (-122.3825, 2.4508) -> (-122.407, 2.4508)
  spline S73 degree 2 poles (-122.407, 2.4508) (-122.4193, 2.4508) (-122.4193, 2.4631) knots 0 0 0 1 1 1
  spline S74 degree 2 poles (-122.4193, 2.4631) (-122.4193, 2.4753) (-122.2723, 2.9406) (-122.2723, 3.2957) knots 0 0 0 1 2 2 2
  spline S75 degree 2 poles (-122.2723, 3.2957) (-122.2723, 3.3937) (-122.3458, 3.4059) knots 0 0 0 1 1 1
  line L398 (-122.3458, 3.4059) -> (-122.2478, 3.6141)
  line L399 (-122.2478, 3.6141) -> (-122.2478, 4.5325)
  line L400 (-122.2478, 4.5325) -> (-122.1254, 4.7896)
  spline S76 degree 2 poles (-122.1254, 4.7896) (-122.0642, 4.9121) (-122.0029, 5.2672) knots 0 0 0 1 1 1
  spline S77 degree 2 poles (-122.0029, 5.2672) (-121.905, 5.3284) (-121.8927, 5.3896) knots 0 0 0 1 1 1
  line L401 (-121.8927, 5.3896) -> (-121.954, 5.4753)
  line L402 (-121.954, 5.4753) -> (-121.8927, 5.6345)
  spline S78 degree 2 poles (-121.8927, 5.6345) (-122.0029, 5.8672) (-122.1621, 5.8672) knots 0 0 0 1 1 1
  line L403 (-122.1621, 5.8672) -> (-122.5295, 5.8672)
  spline S79 degree 2 poles (-122.5295, 5.8672) (-122.5907, 5.8059) (-122.5907, 5.7325) knots 0 0 0 1 1 1
  line L404 (-122.5907, 5.7325) -> (-122.6397, 5.7325)
  spline S80 degree 2 poles (-122.6397, 5.7325) (-122.6764, 5.5243) (-122.8356, 5.4753) knots 0 0 0 1 1 1
  spline S81 degree 2 poles (-122.8356, 5.4753) (-122.8723, 5.2794) (-123.056, 5.2427) knots 0 0 0 1 1 1
  line L405 (-123.056, 5.2427) -> (-123.1907, 5.0223)
  line L406 (-123.1907, 5.0223) -> (-123.2274, 5.0223)
  spline S82 degree 2 poles (-123.2274, 5.0223) (-123.2764, 4.8508) (-123.4111, 4.8508) knots 0 0 0 1 1 1
  spline S83 degree 2 poles (-123.4111, 4.8508) (-123.5703, 4.8508) (-123.754, 5.2917) (-123.754, 5.3162) knots 0 0 0 1 2 2 2
  spline S84 degree 2 poles (-123.754, 5.3162) (-123.754, 5.3529) (-123.7295, 5.3896) knots 0 0 0 1 1 1
  spline S85 degree 2 poles (-123.7295, 5.3896) (-123.6438, 5.7202) (-123.2519, 5.9406) knots 0 0 0 1 1 1
  line L407 (-123.2519, 5.9406) -> (-123.2519, 6.0019)
  spline S86 degree 2 poles (-123.2519, 6.0019) (-123.0805, 6.1733) (-122.9091, 6.2468) knots 0 0 0 1 1 1
  line L408 (-122.9091, 6.2468) -> (-122.9825, 6.2468)
  spline S87 degree 2 poles (-122.9825, 6.2468) (-122.6519, 6.3202) (-122.5417, 6.859) (-122.1989, 6.859) knots 0 0 0 1 2 2 2
  line L409 (-122.1989, 6.859) -> (-122.1131, 6.8223)
  line L410 (-122.1131, 6.8223) -> (-121.9172, 6.9202)
  line L411 (-121.9172, 6.9202) -> (-122.0274, 6.9202)
  line L412 (-122.0274, 6.9202) -> (-121.856, 7.0304)
  line L413 (-121.856, 7.0304) -> (-121.807, 7.0059)
  line L414 (-121.807, 7.0059) -> (-121.6723, 7.1651)
  line L415 (-121.6723, 7.1651) -> (-121.6356, 7.1406)
  spline S88 degree 2 poles (-121.6356, 7.1406) (-121.5499, 7.3611) (-121.2193, 7.3611) knots 0 0 0 1 1 1
  spline S89 degree 2 poles (-121.2193, 7.3611) (-121.1458, 7.3611) (-121.1458, 7.4223) knots 0 0 0 1 1 1
  line L416 (-121.1458, 7.4223) -> (-121.1458, 7.4957)
  line L417 (-121.1458, 7.4957) -> (-121.0846, 7.4957)
  line L418 (-121.0846, 7.4957) -> (-121.1091, 7.5202)
  line L419 (-121.1091, 7.5202) -> (-120.8642, 7.7039)
  spline S90 degree 2 poles (-120.8642, 7.7039) (-120.7417, 7.9121) (-120.4723, 7.9121) knots 0 0 0 1 1 1
  spline S91 degree 2 poles (-120.4723, 7.9121) (-120.3131, 7.9121) (-120.056, 7.7284) (-120.056, 7.6427) knots 0 0 0 1 2 2 2
  spline S92 degree 2 poles (-120.056, 7.6427) (-120.056, 7.5447) (-120.1662, 7.3611) knots 0 0 0 1 1 1
  line L420 (-119.0642, 11.7937) -> (-119.1131, 11.7937)
  line L421 (-119.1131, 11.7937) -> (-119.3948, 11.1937)
  line L422 (-119.3948, 11.1937) -> (-119.4193, 11.2304)
  spline S93 degree 2 poles (-119.4193, 11.2304) (-119.4193, 11.1447) (-119.4927, 11.0835) knots 0 0 0 1 1 1
  line L423 (-119.4927, 11.0835) -> (-119.4927, 11.059)
  spline S94 degree 2 poles (-119.4927, 11.059) (-119.6642, 10.7896) (-119.9091, 10.6672) knots 0 0 0 1 1 1
  line L424 (-119.9091, 10.6672) -> (-119.9703, 10.6917)
  line L425 (-119.9703, 10.6917) -> (-119.9703, 10.6427)
  spline S95 degree 2 poles (-119.9703, 10.6427) (-120.2764, 10.6794) (-120.5948, 10.8508) (-120.754, 11.2549) (-120.8274, 11.4753) knots 0 0 0 1 2 3 3 3
  spline S96 degree 2 poles (-120.8274, 11.4753) (-120.7172, 11.6345) (-120.6438, 11.659) knots 0 0 0 1 1 1
  line L426 (-120.6438, 11.659) -> (-120.5825, 11.8672)
  line L427 (-120.5825, 11.8672) -> (-120.3376, 12.0019)
  line L428 (-120.3376, 12.0019) -> (-120.1907, 12.2957)
  line L429 (-120.1907, 12.2957) -> (-119.9458, 12.4304)
  line L430 (-119.9458, 12.4304) -> (-119.9458, 12.3937)
  line L431 (-119.9458, 12.3937) -> (-119.8111, 12.3325)
  spline S97 degree 2 poles (-119.8111, 12.3325) (-119.7499, 12.357) (-119.7131, 12.3937) (-119.6519, 12.4549) (-119.358, 12.5162) (-119.2846, 12.5651) knots 0 0 0 1 2 3 4 4 4
  line L432 (-119.2846, 12.5651) -> (-119.1989, 12.6141)
  line L433 (-119.1989, 12.6141) -> (-119.1376, 12.6141)
  line L434 (-119.1376, 12.6141) -> (-119.0274, 12.4304)
  line L435 (-119.0274, 12.4304) -> (-119.0274, 12.1978)
  line L436 (-119.0274, 12.1978) -> (-118.9907, 11.9774)
  line L437 (-118.9907, 11.9774) -> (-119.0642, 11.7937)
  line L438 (-119.6397, -5.8634) -> (-119.2968, -5.2879)
  line L439 (-119.2968, -5.2879) -> (-119.2356, -5.3369)
  line L440 (-119.2356, -5.3369) -> (-119.1866, -5.1165)
  line L441 (-119.1866, -5.1165) -> (-118.9172, -4.6512)
  line L442 (-118.9172, -4.6512) -> (-118.7703, -4.59)
  line L443 (-118.7703, -4.59) -> (-118.7458, -4.4553)
  line L444 (-118.7458, -4.4553) -> (-118.5499, -4.2594)
  spline S98 degree 2 poles (-118.5499, -4.2594) (-118.4397, -3.99) (-118.4152, -3.9777) knots 0 0 0 1 1 1
  line L445 (-118.4152, -3.9777) -> (-118.4152, -3.9287)
  spline S99 degree 2 poles (-118.4152, -3.9287) (-118.3785, -3.892) (-118.2193, -3.5369) knots 0 0 0 1 1 1
  spline S100 degree 2 poles (-118.2193, -3.5369) (-118.1213, -3.2798) (-118.0723, -3.2553) knots 0 0 0 1 1 1
  spline S101 degree 2 poles (-118.0723, -3.2553) (-117.9866, -2.8145) (-117.8274, -2.5083) knots 0 0 0 1 1 1
  line L446 (-117.8274, -2.5083) -> (-117.7172, -2.092)
  line L447 (-117.7172, -2.092) -> (-117.7172, -1.9818)
  line L448 (-117.7172, -1.9818) -> (-117.607, -1.8104)
  line L449 (-117.607, -1.8104) -> (-117.3866, -0.7328)
  line L450 (-117.3866, -0.7328) -> (-117.3866, -0.5981)
  spline S102 degree 2 poles (-117.3866, -0.5981) (-117.3131, -0.5369) (-117.3009, -0.3655) knots 0 0 0 1 1 1
  line L451 (-117.3009, -0.3655) -> (-117.154, 0.6019)
  line L452 (-117.154, 0.6019) -> (-116.9703, 0.8468)
  line L453 (-116.9703, 0.8468) -> (-117.0193, 1.0427)
  line L454 (-117.0193, 1.0427) -> (-116.9703, 1.1896)
  line L455 (-116.9703, 1.1896) -> (-116.8601, 1.8264)
  line L456 (-116.8601, 1.8264) -> (-116.7989, 1.9611)
  line L457 (-116.7989, 1.9611) -> (-116.8356, 2.1815)
  line L458 (-116.8356, 2.1815) -> (-116.7989, 2.2427)
  line L459 (-116.7989, 2.2427) -> (-116.6519, 2.8549)
  line L460 (-116.6519, 2.8549) -> (-116.6274, 3.0998)
  line L461 (-116.6274, 3.0998) -> (-116.554, 3.3202)
  line L462 (-116.554, 3.3202) -> (-116.5785, 3.6019)
  line L463 (-116.5785, 3.6019) -> (-116.554, 3.6508)
  line L464 (-116.554, 3.6508) -> (-116.3825, 3.6264)
  line L465 (-116.3825, 3.6264) -> (-116.2356, 4.1284)
  line L466 (-116.2356, 4.1284) -> (-116.2356, 4.3243)
  line L467 (-116.2356, 4.3243) -> (-116.1621, 4.7896)
  line L468 (-116.1621, 4.7896) -> (-116.0519, 4.8264)
  line L469 (-116.0519, 4.8264) -> (-116.0519, 5.0713)
  line L470 (-116.0519, 5.0713) -> (-115.9907, 5.1815)
  line L471 (-115.9907, 5.1815) -> (-115.9907, 5.5366)
  line L472 (-115.9907, 5.5366) -> (-115.7703, 6.1243)
  line L473 (-115.7703, 6.1243) -> (-115.7458, 6.2713)
  line L474 (-115.7458, 6.2713) -> (-115.7948, 6.4059)
  line L475 (-115.7948, 6.4059) -> (-115.6356, 6.7366)
  line L476 (-115.6356, 6.7366) -> (-115.6356, 6.8713)
  line L477 (-115.6356, 6.8713) -> (-115.5866, 7.0304)
  spline S103 degree 2 poles (-115.5866, 7.0304) (-115.8315, 7.2019) (-115.9172, 7.2019) knots 0 0 0 1 1 1
  line L478 (-115.9172, 7.2019) -> (-116.0642, 7.2019)
  line L479 (-116.0642, 7.2019) -> (-116.1621, 7.1406)
  line L480 (-116.1621, 7.1406) -> (-116.3825, 7.2264)
  line L481 (-116.3825, 7.2264) -> (-116.4927, 7.2264)
  line L482 (-116.4927, 7.2264) -> (-116.6029, 7.4835)
  line L483 (-116.6029, 7.4835) -> (-116.9091, 7.5447)
  line L484 (-116.9091, 7.5447) -> (-117.0193, 7.6549)
  line L485 (-117.0193, 7.6549) -> (-117.1295, 7.6549)
  line L486 (-117.1295, 7.6549) -> (-117.2642, 7.8998)
  line L487 (-117.2642, 7.8998) -> (-117.2642, 8.0835)
  line L488 (-117.2642, 8.0835) -> (-117.5458, 8.4631)
  line L489 (-117.5458, 8.4631) -> (-117.3866, 8.6835)
  line L490 (-117.3866, 8.6835) -> (-117.1907, 8.6835)
  spline S104 degree 2 poles (-117.1907, 8.6835) (-117.1785, 8.708) (-117.0438, 8.7692) knots 0 0 0 1 1 1
  line L491 (-117.0438, 8.7692) -> (-117.0193, 8.8794)
  line L492 (-117.0193, 8.8794) -> (-116.9336, 8.8794)
  spline S105 degree 2 poles (-116.9336, 8.8794) (-116.8723, 8.9774) (-116.6764, 9.0998) knots 0 0 0 1 1 1
  line L493 (-116.6764, 9.0998) -> (-116.5172, 9.0998)
  spline S106 degree 2 poles (-116.5172, 9.0998) (-116.2968, 8.9651) (-116.1254, 8.4876) knots 0 0 0 1 1 1
  line L494 (-116.1254, 8.4876) -> (-115.7703, 8.4876)
  line L495 (-115.7703, 8.4876) -> (-115.7091, 8.3529)
  line L496 (-115.7091, 8.3529) -> (-115.6356, 8.4264)
  line L497 (-115.6356, 8.4264) -> (-115.5254, 8.3284)
  line L498 (-115.5254, 8.3284) -> (-115.3785, 8.2917)
  line L499 (-115.3785, 8.2917) -> (-115.2193, 8.2917)
  line L500 (-115.2193, 8.2917) -> (-115.0478, 8.8182)
  line L501 (-115.0478, 8.8182) -> (-115.0234, 9.0264)
  line L502 (-115.0234, 9.0264) -> (-114.9989, 8.9896)
  line L503 (-114.9989, 8.9896) -> (-115.0234, 9.1243)
  line L504 (-115.0234, 9.1243) -> (-114.9376, 9.2345)
  line L505 (-114.9376, 9.2345) -> (-114.9621, 9.4059)
  line L506 (-114.9621, 9.4059) -> (-114.8887, 9.4794)
  spline S107 degree 2 poles (-114.8887, 9.4794) (-114.8152, 9.6876) (-114.7417, 9.7978) knots 0 0 0 1 1 1
  line L507 (-114.7417, 9.7978) -> (-114.8274, 9.8345)
  line L508 (-114.8274, 9.8345) -> (-114.6805, 10.1529)
  line L509 (-114.6805, 10.1529) -> (-114.6438, 10.1162)
  line L510 (-114.6438, 10.1162) -> (-114.607, 10.2141)
  line L511 (-114.607, 10.2141) -> (-114.5825, 10.2141)
  line L512 (-114.5825, 10.2141) -> (-114.5825, 10.3733)
  line L513 (-114.5825, 10.3733) -> (-114.4601, 10.459)
  line L514 (-114.4601, 10.459) -> (-114.3989, 10.7896)
  line L515 (-114.3989, 10.7896) -> (-114.4601, 10.9366)
  line L516 (-114.4601, 10.9366) -> (-114.3009, 11.3162)
  line L517 (-114.3009, 11.3162) -> (-114.1785, 11.3774)
  line L518 (-114.1785, 11.3774) -> (-114.1785, 11.4876)
  line L519 (-114.1785, 11.4876) -> (-113.8846, 11.8549)
  spline S108 degree 2 poles (-113.8846, 11.8549) (-113.7989, 11.9162) (-113.5907, 12.1611) knots 0 0 0 1 1 1
  line L520 (-113.5907, 12.1611) -> (-113.5172, 12.1611)
  line L521 (-113.5172, 12.1611) -> (-113.5172, 12.21)
  spline S109 degree 2 poles (-113.5172, 12.21) (-113.407, 12.2957) (-113.1254, 12.3692) knots 0 0 0 1 1 1
  line L522 (-113.1254, 12.3692) -> (-113.0274, 12.6264)
  line L523 (-113.0274, 12.6264) -> (-112.807, 12.6876)
  line L524 (-112.807, 12.6876) -> (-112.7703, 12.8713)
  line L525 (-112.7703, 12.8713) -> (-112.4887, 12.8345)
  line L526 (-112.4887, 12.8345) -> (-112.4642, 12.9325)
  line L527 (-112.4642, 12.9325) -> (-111.5458, 13.3978)
  line L528 (-111.5458, 13.3978) -> (-111.3376, 13.2876)
  spline S110 degree 2 poles (-111.3376, 13.2876) (-110.8601, 13.3855) (-110.7989, 13.3733) knots 0 0 0 1 1 1
  line L529 (-110.7989, 13.3733) -> (-110.2234, 13.1406)
  line L530 (-110.2234, 13.1406) -> (-110.1376, 12.5162)
  line L531 (-110.1376, 12.5162) -> (-110.0274, 12.0998)
  line L532 (-110.0274, 12.0998) -> (-110.6764, 11.5611)
  line L533 (-110.6764, 11.5611) -> (-111.0193, 11.757)
  line L534 (-111.0193, 11.757) -> (-111.2642, 11.7202)
  line L535 (-111.2642, 11.7202) -> (-111.6682, 11.8182)
  line L536 (-111.6682, 11.8182) -> (-111.6682, 12.1243)
  line L537 (-111.6682, 12.1243) -> (-111.8887, 12.0631)
  line L538 (-111.8887, 12.0631) -> (-112.1336, 12.1243)
  line L539 (-112.1336, 12.1243) -> (-112.207, 12.2957)
  line L540 (-112.207, 12.2957) -> (-112.3295, 12.2345)
  line L541 (-112.3295, 12.2345) -> (-112.354, 12.1611)
  line L542 (-112.354, 12.1611) -> (-112.4642, 12.2713)
  line L543 (-112.4642, 12.2713) -> (-112.4887, 11.9896)
  line L544 (-112.4887, 11.9896) -> (-112.6723, 11.8549)
  spline S111 degree 2 poles (-112.6723, 11.8549) (-112.7825, 11.4998) (-112.9417, 11.3162) knots 0 0 0 1 1 1
  line L545 (-112.9417, 11.3162) -> (-112.9417, 11.2427)
  line L546 (-112.9417, 11.2427) -> (-113.1254, 11.0713)
  line L547 (-113.1254, 11.0713) -> (-113.1621, 10.8141)
  line L548 (-113.1621, 10.8141) -> (-113.3336, 10.7162)
  line L549 (-113.3336, 10.7162) -> (-113.3336, 10.6059)
  line L550 (-113.3336, 10.6059) -> (-113.407, 10.6059)
  spline S112 degree 2 poles (-113.407, 10.6059) (-113.4438, 10.459) (-113.4805, 10.3243) knots 0 0 0 1 1 1
  line L551 (-113.4805, 10.3243) -> (-113.5907, 10.3733)
  line L552 (-113.5907, 10.3733) -> (-113.6642, 10.2141)
  line L553 (-113.6642, 10.2141) -> (-113.6642, 10.1162)
  line L554 (-113.6642, 10.1162) -> (-113.6887, 10.1162)
  line L555 (-113.6887, 10.1162) -> (-113.6642, 10.0182)
  spline S113 degree 2 poles (-113.6642, 10.0182) (-113.9091, 9.6386) (-113.9703, 9.2345) knots 0 0 0 1 1 1
  line L556 (-113.9703, 9.2345) -> (-114.0438, 9.1978)
  line L557 (-114.0438, 9.1978) -> (-114.105, 9.0631)
  line L558 (-114.105, 9.0631) -> (-114.105, 8.8794)
  line L559 (-114.105, 8.8794) -> (-114.1785, 8.9039)
  line L560 (-114.1785, 8.9039) -> (-114.2274, 8.708)
  line L561 (-114.2274, 8.708) -> (-114.3744, 8.4264)
  spline S114 degree 2 poles (-114.3744, 8.4264) (-114.4601, 8.2672) (-114.4601, 8.1447) knots 0 0 0 1 1 1
  line L562 (-114.4601, 8.1447) -> (-114.3989, 7.9611)
  line L563 (-114.3989, 7.9611) -> (-114.2764, 7.8876)
  spline S115 degree 2 poles (-114.2764, 7.8876) (-114.2029, 7.8386) (-114.1172, 7.8386) knots 0 0 0 1 1 1
  line L564 (-114.1172, 7.8386) -> (-113.8968, 7.8264)
  line L565 (-113.8968, 7.8264) -> (-113.7254, 7.6427)
  line L566 (-113.7254, 7.6427) -> (-113.6274, 7.6427)
  line L567 (-113.6274, 7.6427) -> (-113.5662, 7.6672)
  line L568 (-113.5662, 7.6672) -> (-113.4805, 7.6427)
  line L569 (-113.4805, 7.6427) -> (-113.3458, 7.6672)
  line L570 (-113.3458, 7.6672) -> (-113.2723, 7.5692)
  line L571 (-113.2723, 7.5692) -> (-113.1254, 7.6182)
  line L572 (-113.1254, 7.6182) -> (-113.0029, 7.6182)
  line L573 (-113.0029, 7.6182) -> (-113.0029, 7.7284)
  line L574 (-113.0029, 7.7284) -> (-112.8927, 7.7896)
  line L575 (-112.8927, 7.7896) -> (-112.8315, 7.7406)
  line L576 (-112.8315, 7.7406) -> (-112.6968, 7.7896)
  line L577 (-112.6968, 7.7896) -> (-112.6234, 7.6182)
  line L578 (-112.6234, 7.6182) -> (-112.5376, 7.7774)
  line L579 (-112.5376, 7.7774) -> (-112.3907, 7.5815)
  line L580 (-112.3907, 7.5815) -> (-112.2927, 7.7039)
  line L581 (-112.2927, 7.7039) -> (-112.1336, 7.6672)
  line L582 (-112.1336, 7.6672) -> (-112.1336, 7.7284)
  line L583 (-112.1336, 7.7284) -> (-111.8887, 7.7039)
  spline S116 degree 2 poles (-111.8887, 7.7039) (-111.8274, 7.7284) (-111.7295, 7.7651) knots 0 0 0 1 1 1
  line L584 (-111.7295, 7.7651) -> (-111.6315, 7.7162)
  line L585 (-111.6315, 7.7162) -> (-111.4234, 7.7162)
  line L586 (-111.4234, 7.7162) -> (-111.2519, 7.3733)
  line L587 (-111.2519, 7.3733) -> (-111.3009, 7.1896)
  line L588 (-111.3009, 7.1896) -> (-111.4478, 7.1039)
  spline S117 degree 2 poles (-111.4478, 7.1039) (-111.5825, 7.0672) (-111.705, 7.0182) knots 0 0 0 1 1 1
  line L589 (-111.705, 7.0182) -> (-111.7785, 6.908)
  line L590 (-111.7785, 6.908) -> (-111.9866, 6.9325)
  line L591 (-111.9866, 6.9325) -> (-112.1091, 6.8468)
  line L592 (-112.1091, 6.8468) -> (-112.2438, 6.9447)
  line L593 (-112.2438, 6.9447) -> (-112.2927, 6.7855)
  line L594 (-112.2927, 6.7855) -> (-112.4642, 6.7855)
  line L595 (-112.4642, 6.7855) -> (-112.5744, 6.8468)
  line L596 (-112.5744, 6.8468) -> (-112.7336, 6.8468)
  line L597 (-112.7336, 6.8468) -> (-112.8315, 6.8835)
  line L598 (-112.8315, 6.8835) -> (-113.0029, 6.7855)
  line L599 (-113.0029, 6.7855) -> (-113.1254, 6.81)
  line L600 (-113.1254, 6.81) -> (-113.2478, 6.7121)
  line L601 (-113.2478, 6.7121) -> (-113.3825, 6.7978)
  line L602 (-113.3825, 6.7978) -> (-113.456, 6.6631)
  line L603 (-113.456, 6.6631) -> (-113.6029, 6.6631)
  line L604 (-113.6029, 6.6631) -> (-113.6274, 6.7366)
  line L605 (-113.6274, 6.7366) -> (-113.7866, 6.6631)
  line L606 (-113.7866, 6.6631) -> (-114.0682, 6.7366)
  line L607 (-114.0682, 6.7366) -> (-114.4356, 6.6264)
  line L608 (-114.4356, 6.6264) -> (-114.5825, 6.7733)
  line L609 (-114.5825, 6.7733) -> (-114.7907, 6.4917)
  line L610 (-114.7907, 6.4917) -> (-114.9376, 6.4549)
  line L611 (-114.9376, 6.4549) -> (-114.9621, 6.0998)
  line L612 (-114.9621, 6.0998) -> (-114.9989, 6.1243)
  line L613 (-114.9989, 6.1243) -> (-114.9989, 5.9529)
  line L614 (-114.9989, 5.9529) -> (-115.158, 5.6345)
  line L615 (-115.158, 5.6345) -> (-115.0968, 5.5366)
  line L616 (-115.0968, 5.5366) -> (-115.158, 5.3162)
  line L617 (-115.158, 5.3162) -> (-115.158, 4.9366)
  line L618 (-115.158, 4.9366) -> (-115.2438, 4.9611)
  line L619 (-115.2438, 4.9611) -> (-115.2438, 4.7651)
  line L620 (-115.2438, 4.7651) -> (-115.3172, 4.4345)
  spline S118 degree 2 poles (-115.3172, 4.4345) (-115.5009, 4.0672) (-115.5009, 3.8713) knots 0 0 0 1 1 1
  line L621 (-115.5009, 3.8713) -> (-115.4642, 3.6508)
  spline S119 degree 2 poles (-115.4642, 3.6508) (-115.6234, 3.3815) (-115.6356, 3.3202) knots 0 0 0 1 1 1
  line L622 (-115.6356, 3.3202) -> (-115.5621, 3.1611)
  line L623 (-115.5621, 3.1611) -> (-115.6601, 3.0631)
  line L624 (-115.6601, 3.0631) -> (-115.6601, 2.9284)
  line L625 (-115.6601, 2.9284) -> (-115.5621, 2.8182)
  line L626 (-115.5621, 2.8182) -> (-115.5989, 2.6835)
  line L627 (-115.5989, 2.6835) -> (-115.5621, 2.5733)
  line L628 (-115.5621, 2.5733) -> (-115.7703, 2.3162)
  line L629 (-115.7703, 2.3162) -> (-115.7091, 2.157)
  line L630 (-115.7091, 2.157) -> (-115.7948, 1.9611)
  line L631 (-115.7948, 1.9611) -> (-115.856, 1.3733)
  line L632 (-115.856, 1.3733) -> (-115.9172, 1.2631)
  line L633 (-115.9172, 1.2631) -> (-115.8805, 1.1651)
  line L634 (-115.8805, 1.1651) -> (-116.0152, 0.9815)